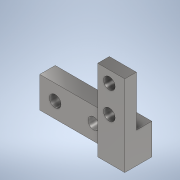
# Autodesk Inventor part: Soporte Switch X Izq
Saved by Autodesk Inventor 2021 (Build 250183000, 183)
## iProperties
Created: 2023-01-30
Part Number: Soporte Switch X Izq
Material: Acero, fundido
Document SubType Name: Modeling
Designer: Diego.labarca
Density: 7.85 g/cm^3
Appearance: Semipulido
Author: Diego.labarca
Autodesk Inventor part; units mm, degrees
ref_plane "YZ Plane" through (0, 0, 0) normal (1, 0, 0) x (0, 1, 0)
ref_plane "XZ Plane" through (0, 0, 0) normal (0, 1, 0) x (-1, 0, 0)
ref_plane "XY Plane" through (0, 0, 0) normal (0, 0, 1) x (1, 0, 0)
sketch "Boceto1" plane through (0, 0, 0) normal (0, 0, 1) x (1, 0, 0)
  line L0 (-15.9664, 2.6415) -> (9.0336, 2.6415)
  line L1 (9.0336, 2.6415) -> (9.0336, -5.3585)
  line L2 (9.0336, -5.3585) -> (-15.9664, -5.3585)
  line L3 (-15.9664, -5.3585) -> (-15.9664, 2.6415)
  circle A0 centre (-11.9664, -1.3585) radius 1.5
  circle A1 centre (-1.9664, -1.3585) radius 1.5
  point P0 (0, 0)
  dimension "d0" = 3
  dimension "d1" = 3
  dimension "d2" = 25
  dimension "d3" = 8
  dimension "d4" = 10
  dimension "d8" = 4
  dimension "d9" = 4
  dimension "d10" = 4
  constraints: 8 end point, 2 centre point, 2 parallel, 1 horizontal, 1 perpendicular
  measures "d0" diameter of A0
  measures "d1" diameter of A1
  measures "d2" distance of L0.start L0.end
  measures "d3" distance of L0.end L1.end
  measures "d4" distance of A0.centre A1.centre
  measures "d8" distance from line of L3 A0.centre
  measures "d9" distance from line of L0 A1.centre
  measures "d10" distance from line of L0 A0.centre
extrude "Extrusión1" add sketch "Boceto1" along normal blind 4
sketch "Boceto2" plane through (0, 0, 4) normal (0, 0, 1) x (1, 0, 0)
  line L0 (-15.9664, -5.3585) -> (9.0336, -5.3585) projected
  line L1 (9.0336, -5.3585) -> (2.0336, -5.3585)
  line L2 (2.0336, -5.3585) -> (2.0336, 15.6415)
  line L3 (2.0336, 15.6415) -> (9.0336, 15.6415)
  line L4 (9.0336, 15.6415) -> (9.0336, -5.3585)
  point P0 (0, 0)
  dimension "d11" = 7
  dimension "d12" = 21
  constraints: 8 end point, 2 parallel, 1 horizontal, 1 perpendicular
  measures "d11" distance of L2.end L3.end
  measures "d12" distance of L1.end L2.end
extrude "Extrusión2" add sketch "Boceto2" along normal blind 3
sketch "Boceto3" plane through (0, 0, 7) normal (0, 0, 1) x (1, 0, 0)
  circle A0 centre (5.0336, 5.6415) radius 1.5
  circle A1 centre (5.0336, 12.6415) radius 1.5
  line L0 (2.0336, 2.6415) -> (-15.9664, 2.6415) projected
  line L1 (2.0336, 15.6415) -> (2.0336, -5.3585) projected
  point P0 (0, 0)
  dimension "d15" = 7
  dimension "d16" = 3
  dimension "d17" = 3
  dimension "d18" = 3
  dimension "d19" = 3
  dimension "d20" = 3
  constraints: 2 centre point
  measures "d15" distance of A1.centre A0.centre
  measures "d16" distance from line of A0.centre L0
  measures "d17" distance from line of L1 A1.centre
  measures "d18" distance from line of L1 A0.centre
  measures "d19" diameter of A1
  measures "d20" diameter of A0
extrude "Extrusión3" cut sketch "Boceto3" against normal up to surface (3 mm away)
equation "\"d1\" = d0"
equation "\"d9\" = 0.5 * d3"
equation "\"d10\" = d9"
equation "\"d18\" = d17"
equation "\"d20\" = d19"
